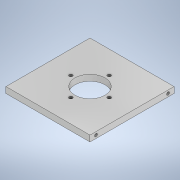
# Autodesk Inventor part: 상판
Saved by Autodesk Inventor 2020.2 (Build 242310000, 310)
## iProperties
Created: 2020-03-28
Part Number: 상판
Material: Aluminum 6061-AHC
Document SubType Name: Modeling
Designer: introbot
Density: 2.7 g/cm^3
Appearance: Aluminum - Dark
Mass: 129.296 g
Surface Area: 133.564 cm^2
Volume: 47.8876 cm^3
Author: introbot
Autodesk Inventor part; units mm, degrees
ref_plane "YZ Plane" through (0, 0, 0) normal (1, 0, 0) x (0, 1, 0)
ref_plane "XZ Plane" through (0, 0, 0) normal (0, 1, 0) x (-1, 0, 0)
sketch "Sketch1" plane through (0, 0, 0) normal (0, 1, 0) x (-1, 0, 0)
  line L0 (35, 35) -> (-35, 35)
  line L1 (-35, 35) -> (-35, -35)
  line L2 (-35, -35) -> (35, -35)
  line L3 (35, -35) -> (35, 35)
  line L4 (0, -49) -> (0, 49) projected
  line L5 (49, 0) -> (-49, 0) projected
  point P0 (0, 0)
  dimension "d0" = 70
  dimension "d1" = 70
  dimension "d2" = 70
  constraints: 8 end point, 2 parallel, 1 horizontal, 1 perpendicular, 2 other
  measures "d0" distance of L2.end L0.start
  measures "d1" distance of L0.start L0.end
  measures "d2" distance of L1.end L2.end
extrude "Extrusion1" add sketch "Sketch1" along normal blind 5
sketch "Sketch2" plane through (35, 0, 35) normal (1, 0, 0) x (0, 0, -1)
  line L0 (0, 0) -> (70, 0) projected
  line L1 (70, 0) -> (70, 5) projected
  line L2 (35, 0) -> (35, 5)
  line L3 (0, 5) -> (70, 5) projected
  point P0 (65, 2.5)
  point P1 (5, 2.5)
  dimension "d5" = 2.5
  dimension "d6" = 5
  constraints: 2 end point, 1 midpoint, 1 symmetric about line
  measures "d5" distance from line of L0 point (65, 2.5)
  measures "d6" distance from line of L1 point (65, 2.5)
hole "Hole1" at (35, 2.5, -30) at (35, 2.5, 30) direction (-1, 0, 0) diameter 2.459 depth 8.8 tip angle 118 thread size "M3x0.5" class "6H" standard "ANSI Metric M Profile"
sketch "Sketch3" plane through (0, 5, 0) normal (0, 1, 0) x (1, 0, 0)
  point P0 (0, 0)
  point P1 (0, 0)
  constraints: 1 coincident
hole "Hole2" at (0, 5, 0) direction (0, -1, 0) diameter 25 depth 10 tip angle 118
sketch "Sketch4" plane through (0, 5, 0) normal (0, 1, 0) x (1, 0, 0)
  point P0 (0, 0)
  point P1 (16, 0)
  point P2 (0, 16)
  point P3 (-16, 0)
  point P4 (0, -16)
  dimension "d21" = 16
  dimension "d24" = 360
  constraints: 5 other
  measures "d21" distance of point (0, 0) point (16, 0)
sketch "Sketch5" plane through (0, 5, 0) normal (0, 1, 0) x (1, 0, 0)
  point P0 (0, 0)
hole "Hole3" at (-16, 5, 0) at (0, 5, -16) at (0, 5, 16) at (16, 5, 0) direction (0, -1, 0) diameter 2.85 depth 10.4 tip angle 118 thread size "M3.5x0.6" class "6H" standard "ANSI Metric M Profile"
ref_plane "Work Plane2" through (0, 0, -35) normal (-1, 0, 0) x (0, 0, 1)
mirror "Mirror2" about plane through (0, 0, -35) normal (-1, 0, 0) of "Hole1"
body "Solid1"
